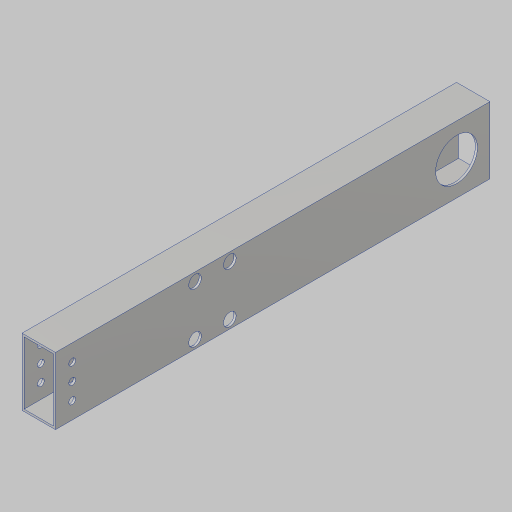
# Autodesk Inventor part: CL3-003
Saved by Autodesk Inventor 2023.5 (Build 275446000, 446)
## iProperties
RuleStatus: InUse
Created: 2025-01-28
Part Number: CL3-003
Material: Aluminum 6061
Document SubType Name: Modeling
Designer: slick
Mass: 304.185 g
Surface Area: 718.547 cm^2
Volume: 112.661 cm^3
Density: 2.7 g/cm^3
Appearance: Aluminum - Flat
AfterDocNew0: SHOW
AfterDocOpen0: SHOW
Author: slick
Autodesk Inventor part; units mm, degrees
ref_plane "YZ Plane" through (0, 0, 0) normal (1, 0, 0) x (0, 1, 0)
ref_plane "XZ Plane" through (0, 0, 0) normal (0, 1, 0) x (-1, 0, 0)
ref_plane "XY Plane" through (0, 0, 0) normal (0, 0, 1) x (1, 0, 0)
sketch "Sketch1" plane through (0, 0, 0) normal (0, 0, 1) x (1, 0, 0)
  line L0 (-12.7, -25.4) -> (12.7, -25.4)
  line L1 (12.7, -25.4) -> (12.7, 25.4)
  line L2 (12.7, 25.4) -> (-12.7, 25.4)
  line L3 (-12.7, 25.4) -> (-12.7, -25.4)
  line L4 (-12.7, -25.4) -> (12.7, 25.4) construction
  line L5 (12.7, -25.4) -> (-12.7, 25.4) construction
  line L6 (-11.1125, 23.8125) -> (11.1125, 23.8125)
  line L7 (11.1125, 23.8125) -> (11.1125, -23.8125)
  line L8 (11.1125, -23.8125) -> (-11.1125, -23.8125)
  line L9 (-11.1125, -23.8125) -> (-11.1125, 23.8125)
  point P0 (0, 0)
  dimension "width" = 25.4
  dimension "height" = 50.8
  dimension "thickness" = 1.5875
  constraints: 20 end point, 4 parallel, 2 midpoint, 2 perpendicular, 1 horizontal, 3 other
  measures "width" distance of L2.end L1.end
  measures "height" distance of L1.end L0.end
  measures "thickness" distance between parallel lines of L2 L6
extrude "Extrusion1" add sketch "Sketch1" along normal mid plane 330.2
sketch "Sketch3" plane through (12.7, -25.4, -165.1) normal (1, 0, 0) x (0, 0, -1)
  circle A0 centre (-25.4, 25.4) radius 15.875
  line L0 (0, 50.8) -> (0, 0) projected
  point P0 (-165.1, 25.4)
  dimension "d8" = 31.75
  dimension "d9" = 25.4
  constraints: 1 centre point, 1 horizontal alignment
  measures "d8" diameter of A0
  measures "d9" distance from line of L0 A0.centre
extrude "Extrusion3" cut sketch "Sketch3" against normal up to surface (1.5875 mm away)
sketch "Sketch4" plane through (12.7, -25.4, 165.1) normal (1, 0, 0) x (0, 0, -1)
  circle A0 centre (304.8, 25.4) radius 15.875 construction
  line L0 (330.2, 50.8) -> (330.2, 0) construction
  line L1 (330.2, 0) -> (0, 0) construction
  line L2 (0, 0) -> (0, 50.8) construction
  line L3 (0, 50.8) -> (330.2, 50.8) construction
  point P0 (165.1, 25.4)
  point P1 (12.7, 25.4)
  point P2 (12.7, 12.7)
  point P3 (12.7, 38.1)
  point P4 (0, 25.4)
  dimension "d12" = 12.7
  dimension "d13" = 12.7
  dimension "d14" = 12.7
  constraints: 2 vertical alignment, 1 horizontal alignment, 1 midpoint
  measures "d12" distance from line of L2 point (12.7, 25.4)
  measures "d13" distance of point (12.7, 25.4) point (12.7, 38.1)
  measures "d14" distance of point (12.7, 12.7) point (12.7, 25.4)
hole "Hole1" at (12.7, 0, 152.4) at (12.7, -12.7, 152.4) at (12.7, 12.7, 152.4) direction (-1, 0, 0) diameter 5.1054 end through all clearance for "Flat Head Machine Screw (82)" size "#10" standard "Ansi Unified Screw Threads"
sketch "Sketch6" plane through (-12.7, -25.4, 165.1) normal (-1, 0, 0) x (0, 0, 1)
  line L0 (-330.2, 0) -> (0, 0) construction
  line L1 (0, 0) -> (-152.4, 0) construction
  circle A0 centre (-12.7, 12.7) radius 2.5527 construction
  circle A1 centre (-12.7, 25.4) radius 2.5527 construction
  circle A2 centre (-12.7, 38.1) radius 2.5527 construction
  line L2 (-330.2, 0) -> (-330.2, 50.8) construction
  line L3 (-330.2, 50.8) -> (0, 50.8) construction
  line L4 (0, 50.8) -> (0, 0) construction
  line L5 (0, 0) -> (-330.2, 0) construction
  circle A3 centre (-12.7, 12.7) radius 2.5527 construction
  circle A4 centre (-12.7, 25.4) radius 2.5527 construction
  circle A5 centre (-12.7, 38.1) radius 2.5527 construction
  line L6 (-330.2, 0) -> (-330.2, 50.8) construction
  line L7 (-330.2, 50.8) -> (0, 50.8) construction
  line L8 (0, 50.8) -> (0, 0) construction
  line L9 (0, 0) -> (-330.2, 0) construction
  line L10 (-152.4, 0) -> (-50.8, 146.1832) construction
  line L11 (0, 0) -> (0, 203.2) construction
  line L12 (0, 203.2) -> (-50.8, 203.2) construction
  line L13 (-50.8, 203.2) -> (-50.8, 146.1832) construction
  circle A6 centre (-106.0668, 44.4119) radius 4.8006 construction
  circle A7 centre (-132.494, 6.3881) radius 4.8006 construction
  line L14 (-106.0668, 44.4119) -> (-132.494, 6.3881) construction
  circle A8 centre (-12.7, 12.7) radius 2.5527 construction
  circle A9 centre (-12.7, 25.4) radius 2.5527 construction
  circle A10 centre (-12.7, 38.1) radius 2.5527 construction
  line L15 (-330.2, 0) -> (-330.2, 50.8) construction
  line L16 (-330.2, 50.8) -> (0, 50.8) construction
  line L17 (0, 50.8) -> (0, 0) construction
  line L18 (0, 0) -> (-330.2, 0) construction
  line L19 (0, 1.5875) -> (-330.2, 1.5875) construction
  line L20 (-330.2, 49.2125) -> (0, 49.2125) construction
  point P0 (-165.1, 25.4)
  dimension "d35" = 152.4
  dimension "d36" = 55.2
  dimension "d37" = 203.2
  dimension "d38" = 50.8
  dimension "d39" = 9.6012
  dimension "d40" = 12.7
  constraints: 12 end point, 2 centre point, 2 coincident, 2 perpendicular, 2 point on line, 2 tangent, 1 equal radius, 1 parallel
  measures "d35" distance of L0.end L1.end
  measures "d36" angle of L0 L10
  measures "d37" distance of L0.end L11.end
  measures "d38" distance of L11.end L12.end
  measures "d39" diameter of A6
  measures "d40" distance between parallel lines of L14 L10
hole "Hole3" at (-12.7, 19.0119, 59.0332) at (-12.7, -19.0119, 32.606) direction (1, 0, 0) diameter 9.525 end through all
sketch "Sketch7" plane through (12.7, -25.4, 165.1) normal (1, 0, 0) x (0, 0, -1)
  circle A0 centre (106.0668, 44.4119) radius 4.7625 construction
  circle A1 centre (132.494, 6.3881) radius 4.7625 construction
  circle A2 centre (12.7, 12.7) radius 2.5527 construction
  circle A3 centre (12.7, 25.4) radius 2.5527 construction
  circle A4 centre (12.7, 38.1) radius 2.5527 construction
  circle A5 centre (304.8, 25.4) radius 15.875 construction
  line L0 (330.2, 50.8) -> (0, 50.8) construction
  line L1 (0, 0) -> (0, 50.8) construction
  line L2 (330.2, 0) -> (0, 0) construction
  line L3 (330.2, 50.8) -> (330.2, 0) construction
  line L4 (0, 1.5875) -> (330.2, 1.5875) construction
  line L5 (0, 49.2125) -> (330.2, 49.2125) construction
  line L6 (0, 50.8) -> (152.4, 50.8) construction
  line L7 (330.2, 50.8) -> (0, 50.8) construction
  line L8 (0, 50.8) -> (0, -152.4) construction
  line L9 (0, -152.4) -> (50.8, -152.4) construction
  line L10 (50.8, -152.4) -> (50.8, -95.3832) construction
  line L11 (152.4, 50.8) -> (50.8, -95.3832) construction
  circle A6 centre (132.494, 44.4119) radius 4.8006 construction
  circle A7 centre (106.0668, 6.3881) radius 4.8006 construction
  line L12 (106.0668, 6.3881) -> (132.494, 44.4119) construction
  point P0 (165.1, 25.4)
  dimension "d48" = 152.4
  dimension "d49" = 203.2
  dimension "d50" = 50.8
  dimension "d51" = 55.2
  dimension "d52" = 9.6012
  dimension "d53" = 12.7
  constraints: 12 end point, 2 centre point, 2 coincident, 2 perpendicular, 2 point on line, 2 tangent, 1 equal radius, 1 parallel
  measures "d48" distance of L0.end L6.end
  measures "d49" distance of L0.end L8.end
  measures "d50" distance of L8.end L9.end
  measures "d51" angle of L6 L11
  measures "d52" diameter of A7
  measures "d53" distance between parallel lines of L12 L11
hole "Hole4" at (12.7, -19.0119, 59.0332) at (12.7, 19.0119, 32.606) direction (-1, 0, 0) diameter 9.525 end through all
equation "\"d14\" = d13"
body "Solid1"
